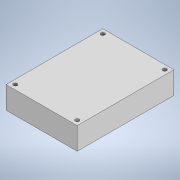
# Autodesk Inventor part: Relay Board
Saved by Autodesk Inventor 2020 (Build 240168000, 168)
## iProperties
Created: 2020-01-26
Part Number: Relay Board
Material: Generic
Document SubType Name: Modeling
Designer: holtat
Density: 1 g/cm^3
Appearance: Default
Author: holtat
Autodesk Inventor part; units mm, degrees
ref_plane "YZ Plane" through (0, 0, 0) normal (1, 0, 0) x (0, 1, 0)
ref_plane "XZ Plane" through (0, 0, 0) normal (0, 1, 0) x (-1, 0, 0)
ref_plane "XY Plane" through (0, 0, 0) normal (0, 0, 1) x (1, 0, 0)
sketch "Sketch1" plane through (0, 0, 0) normal (0, 1, 0) x (-1, 0, 0)
  line L0 (27.559, -37.465) -> (-27.559, -37.465)
  line L1 (-27.559, -37.465) -> (-27.559, 37.465)
  line L2 (-27.559, 37.465) -> (27.559, 37.465)
  line L3 (27.559, 37.465) -> (27.559, -37.465)
  circle A0 centre (24.003, -33.909) radius 1.4605
  circle A1 centre (-24.003, -33.909) radius 1.4605
  circle A2 centre (-24.003, 33.909) radius 1.4605
  circle A3 centre (24.003, 33.909) radius 1.4605
  point P0 (0, 0)
  point P1 (0, -37.465)
  point P2 (27.559, 0)
  dimension "d0" = 55.118
  dimension "d1" = 74.93
  dimension "d2" = 2.921
  dimension "d3" = 3.556
  dimension "d4" = 3.556
  dimension "d5" = 3.556
  dimension "d6" = 3.556
  constraints: 8 end point, 4 centre point, 3 equal radius, 3 horizontal alignment, 3 vertical alignment, 2 midpoint, 2 parallel, 1 horizontal, 1 perpendicular
  measures "d0" distance of L0.start L0.end
  measures "d1" distance of L2.end L0.start
  measures "d2" diameter of A0
  measures "d3" distance from line of L3 A0.centre
  measures "d4" distance from line of L0 A0.centre
  measures "d5" distance from line of L1 A1.centre
  measures "d6" distance from line of L2 A2.centre
extrude "Extrusion1" add sketch "Sketch1" along normal blind 17.272
equation "\"d5\" = d3"
equation "\"d6\" = d4"
body "Solid1"
